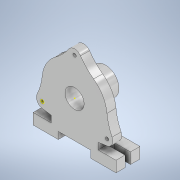
# Autodesk Inventor part: compressor certo certinho msmo
Saved by Autodesk Inventor 2022 (Build 260153000, 153)
## iProperties
Created: 2023-07-28
Part Number: compressor certo certinho msmo
Material: Aluminum 6061-AHC
Document SubType Name: Modeling
Designer: SENAI
Density: 2.7 g/cm^3
Appearance: Aluminum - Dark
Mass: 923.678 g
Surface Area: 662.557 cm^2
Volume: 342.103 cm^3
Author: SENAI
Autodesk Inventor part; units mm, degrees
ref_plane "YZ Plane" through (0, 0, 0) normal (1, 0, 0) x (0, 1, 0)
ref_plane "XZ Plane" through (0, 0, 0) normal (0, 1, 0) x (-1, 0, 0)
ref_plane "XY Plane" through (0, 0, 0) normal (0, 0, 1) x (1, 0, 0)
sketch "Sketch1" plane through (0, 0, 0) normal (0, 0, 1) x (1, 0, 0)
  arc A0 (11.146, 58.6503) -> (-11.146, 58.6503) centre (0, 65.675) ccw
  arc A1 (-56.3657, -19.6724) -> (-45.2196, -38.9779) centre (-56.8762, -32.8375) ccw
  arc A2 (45.2196, -38.9779) -> (56.3657, -19.6724) centre (56.8762, -32.8375) ccw
  circle A3 centre (0, 68.85) radius 3
  circle A4 centre (-59.4093, -34.3) radius 3
  circle A5 centre (59.6258, -34.425) radius 3
  arc A6 (-11.146, 58.6503) -> (-56.3657, -19.6724) centre (0, 0) ccw
  arc A7 (-45.2196, -38.9779) -> (45.2196, -38.9779) centre (0, 0) ccw
  arc A8 (56.3657, -19.6724) -> (11.146, 58.6503) centre (0, 0) ccw
  line L0 (0, 0) -> (-59.4093, -34.3)
  dimension "d4" = 26.35
  dimension "d5" = 26.35
  dimension "d6" = 26.35
  dimension "d13" = 6
  dimension "d14" = 6
  dimension "d15" = 6
  dimension "d60" = 68.6
  constraints: 12 point on circle, 9 centre point, 5 coincident, 2 end point
  measures "d4" diameter of A0
  measures "d5" diameter of A1
  measures "d6" diameter of A2
  measures "d13" diameter of A3
  measures "d14" diameter of A4
  measures "d15" diameter of A5
  measures "d60" distance of L0.start L0.end
extrude "Extrusion1" add sketch "Sketch1" along normal blind 16.5
fillet "Fillet1" radius 100 6 edges at (-11.146, 58.6503, 8.25) (11.146, 58.6503, 8.25) (45.2196, -38.9779, 8.25) (56.3657, -19.6724, 8.25) (-45.2196, -38.9779, 8.25) (-56.3657, -19.6724, 8.25)
sketch "Sketch2" plane through (0, 0, 0) normal (0, 0, -1) x (-1, 0, 0)
  line L0 (0, -67.2336) -> (30, -67.2336)
  line L1 (30, -67.2336) -> (30, -80.2336)
  line L2 (30, -80.2336) -> (76, -80.2336)
  line L3 (76, -80.2336) -> (76, -60.2336)
  line L4 (76, -60.2336) -> (43, -60.2336)
  line L5 (43, -60.2336) -> (43, -48.2336)
  line L6 (0, -67.2336) -> (-30, -67.2336)
  line L7 (-30, -67.2336) -> (-30, -80.2336)
  line L8 (-30, -80.2336) -> (-76, -80.2336)
  line L9 (-76, -80.2336) -> (-76, -60.2336)
  line L10 (-76, -60.2336) -> (-43, -60.2336)
  line L11 (-43, -60.2336) -> (-43, -48.2336)
  arc A0 (-24.4518, -54.4628) -> (-57.8696, -45.975) centre (-65.4096, -145.6903) ccw projected
  line L12 (-43, -48.2336) -> (43, -48.2336)
  point P0 (0, 0)
  dimension "d19" = 30
  dimension "d20" = 13
  dimension "d21" = 46
  dimension "d22" = 20
  dimension "d23" = 33
  dimension "d24" = 12
  dimension "d26" = 13
  dimension "d27" = 46
  dimension "d28" = 20
  dimension "d29" = 33
  dimension "d30" = 12
  constraints: 26 end point, 9 perpendicular, 2 horizontal, 1 point on circle, 1 vertical
  measures "d19" distance of L0.start L0.end
  measures "d20" distance of L0.end L1.end
  measures "d21" distance of L1.end L2.end
  measures "d22" distance of L2.end L3.end
  measures "d23" distance of L3.end L4.end
  measures "d24" distance of L4.end L5.end
  measures "d26" distance of L6.end L7.end
  measures "d27" distance of L7.end L8.end
  measures "d28" distance of L8.end L9.end
  measures "d29" distance of L9.end L10.end
  measures "d30" distance of L10.end L11.end
extrude "Extrusion2" add sketch "Sketch2" against normal blind 16.5
sketch "Sketch3" plane through (0, 0, 0) normal (0, 0, -1) x (-1, 0, 0)
  line L0 (-76, -60.2336) -> (76, -60.2336)
  line L1 (76, -60.2336) -> (76, -80.2336) projected
  line L2 (76, -60.2336) -> (76, -80.2336)
  line L3 (30, -67.2336) -> (30, -80.2336) projected
  line L4 (76, -80.2336) -> (30, -80.2336)
  line L5 (30, -80.2336) -> (30, -67.2336)
  line L6 (-30, -67.2336) -> (30, -67.2336) projected
  line L7 (30, -67.2336) -> (-30, -67.2336)
  line L8 (-30, -67.2336) -> (-30, -80.2336) projected
  line L9 (-30, -67.2336) -> (-30, -80.2336)
  line L10 (-30, -80.2336) -> (-76, -80.2336) projected
  line L11 (-30, -80.2336) -> (-76, -80.2336)
  line L12 (-76, -80.2336) -> (-76, -60.2336) projected
  line L13 (-76, -80.2336) -> (-76, -60.2336)
  point P0 (0, 0)
  constraints: 16 end point, 5 collinear, 2 perpendicular
extrude "Extrusion3" add sketch "Sketch3" along normal blind 27.5
sketch "Sketch4" plane through (-76, -80.2336, 16.5) normal (-1, 0, 0) x (0, 0, 1)
  line L0 (0, 20) -> (-44, 20) projected
  line L1 (-16.5, 20) -> (-16.5, 0)
  line L2 (0, 0) -> (-44, 0) projected
  line L3 (-16.5, 20) -> (3.5, 20) construction
  line L4 (-16.5, 0) -> (-26.5, 0)
  line L5 (-26.5, 0) -> (-26.5, 20)
  line L6 (-26.5, 20) -> (-16.5, 20)
  point P0 (-16.5, 80.2336)
  point P1 (-26.5, 0)
  dimension "d35" = 90
  dimension "d36" = 10
  constraints: 10 end point, 4 perpendicular, 2 point on line, 1 horizontal
  measures "d35" angle of L1 L3
  measures "d36" distance of L1.end L4.end
sketch "Sketch5" plane through (76, -80.2336, 16.5) normal (1, 0, 0) x (0, 0, -1)
  line L0 (16.5, 20) -> (0, 20) projected
  line L1 (16.5, 20) -> (16.5, 0)
  line L2 (0, 0) -> (44, 0) projected
  line L3 (16.5, 0) -> (26.5, 0)
  line L4 (26.5, 0) -> (26.5, 20)
  line L5 (0, 20) -> (44, 20) projected
  line L6 (26.5, 20) -> (16.5, 20)
  point P0 (16.5, 80.2336)
  dimension "d37" = 10
  dimension "d38" = 20
  constraints: 8 end point, 2 perpendicular, 1 point on line, 1 vertical
  measures "d37" distance of L1.end L3.end
  measures "d38" distance of L3.end L4.end
extrude "Extrusion4" cut sketch "Sketch5" against normal blind 30
extrude "Extrusion5" cut sketch "Sketch4" against normal blind 30
sketch "Sketch6" plane through (0, 0, 0) normal (0, 0, -1) x (-1, 0, 0)
  circle A0 centre (0, 0) radius 25
  dimension "d43" = 50
  constraints: 1 centre point, 1 coincident
  measures "d43" diameter of A0
sketch "Sketch7" plane through (0, 0, 0) normal (0, 0, -1) x (-1, 0, 0)
  line L0 (-43, -60.2336) -> (43, -60.2336) projected
  line L1 (0, -60.2336) -> (-5.5, -60.2336)
  line L2 (-5.5, -60.2336) -> (-5.5, -41.2206)
  line L3 (-5.5, -41.2206) -> (5.5, -41.2206)
  line L4 (5.5, -41.2206) -> (5.5, -60.2336)
  line L5 (0, -60.2336) -> (5.5, -60.2336)
  line L6 (-5.5, -41.2206) -> (-5.5, -24.0559)
  line L7 (-5.5, -24.0559) -> (5.5, -24.0559)
  line L8 (5.5, -24.0559) -> (5.5, -41.2206)
  point P0 (0, 0)
  dimension "d45" = 5.5
  dimension "d46" = 19.013
  dimension "d47" = 11
  constraints: 16 end point, 5 perpendicular, 2 point on line, 1 collinear, 1 midpoint, 1 vertical
  measures "d45" distance of L1.start L1.end
  measures "d46" distance of L1.end L2.end
  measures "d47" distance of L2.end L3.end
extrude "Extrusion6" add sketch "Sketch7" along normal blind 27.5
chamfer "Chamfer1" distance 12 angle 45 1 edges at (0, -24.0559, -27.5)
fillet "Fillet2" radius 60 1 edges at (0, -36.0559, -27.5)
extrude "Extrusion7" add sketch "Sketch6" along normal blind 40
sketch "Sketch8" plane through (0, 0, -40) normal (0, 0, -1) x (-1, 0, 0)
  circle A0 centre (0, 0) radius 17.5
  dimension "d56" = 35
  constraints: 1 centre point, 1 coincident
  measures "d56" diameter of A0
extrude "Extrusion8" cut sketch "Sketch8" against normal through all
sketch "Sketch9" plane through (0, 0, 16.5) normal (0, 0, 1) x (1, 0, 0)
  circle A0 centre (-59.4093, -34.3) radius 3 projected
  point P0 (0, 0)
body "Solid1"
